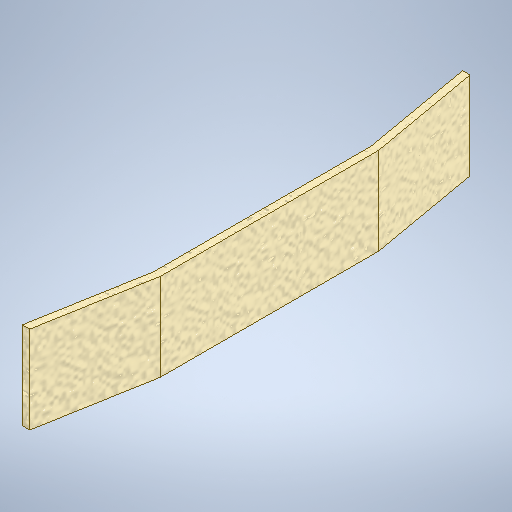
# Autodesk Inventor part: guia
Saved by Autodesk Inventor 2025.2 (Build 292293000, 293)
## iProperties
Created: 2025-11-13
Part Number: guia
Material: Genérico
Document SubType Name: Modeling
Designer: Dax
Density: 1 g/cm^3
Appearance: Fino - Crema
Author: Dax
Autodesk Inventor part; units mm, degrees
ref_plane "YZ Plane" through (0, 0, 0) normal (1, 0, 0) x (0, 1, 0)
ref_plane "XZ Plane" through (0, 0, 0) normal (0, 1, 0) x (-1, 0, 0)
ref_plane "XY Plane" through (0, 0, 0) normal (0, 0, 1) x (1, 0, 0)
sketch "Boceto1" plane through (0, 0, 0) normal (0, 1, 0) x (-1, 0, 0)
  line L0 (-382.6667, -300) -> (-382.6667, -100)
  line L1 (-382.6667, -300) -> (-382.6667, -233.3333)
  line L2 (-382.6667, -233.3333) -> (-382.6667, -300)
  line L3 (-382.6667, -300) -> (-364.7679, -401.509)
  line L4 (-382.6667, -300) -> (-382.6667, -100)
  line L5 (-382.6667, -100) -> (-364.7679, 1.509)
  line L6 (-376, -300) -> (-376, -100)
  line L7 (-376.1013, -298.8423) -> (-357.9984, -401.509)
  line L8 (-376.1013, -101.1577) -> (-357.9984, 1.509)
  line L9 (-357.9984, 1.509) -> (-364.7679, 1.509)
  line L10 (-357.9984, -401.509) -> (-364.7679, -401.509)
  point P0 (0, 0)
  point P1 (-376, -299.4167)
  point P2 (-376, -100.5833)
  dimension "d14" = 200
  constraints: 22 end point, 4 parallel, 1 horizontal, 1 point on line
  measures "d14" distance of L0.start L0.end
extrude "Extrusión1" add sketch "Boceto1" along normal blind 80
